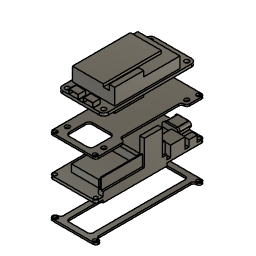
Air_Sensor_Frame (Autodesk Fusion 360 design; units mm, degrees)
Autodesk Fusion 360 part; units mm, degrees
sketch "Sketch1" plane through (0, 0, 0) normal (0, 0, 1) x (1, 0, 0)
  line L0 (-5.5, 4) -> (16.9, 4)
  line L1 (18.4, 2.5) -> (18.4, -54.5)
  line L2 (16.9, -56) -> (-5.5, -56)
  line L3 (-7, -54.5) -> (-7, 2.5)
  line L4 (17.9, 2.5) -> (17.9, 2.5002)
  circle A0 centre (-5.5, 2.5) radius 1
  circle A1 centre (16.9, 2.5) radius 1
  circle A2 centre (16.9, -54.5) radius 1
  circle A3 centre (-5.5, -54.5) radius 1
  line L5 (17.9, 2.5002) -> (17.9, 2.4998)
  arc A4 (-5.5, 4) -> (-7, 2.5) centre (-5.5, 2.5) ccw
  arc A5 (18.4, 2.5) -> (16.9, 4) centre (16.9, 2.5) ccw
  arc A6 (16.9, -56) -> (18.4, -54.5) centre (16.9, -54.5) ccw
  arc A7 (-7, -54.5) -> (-5.5, -56) centre (-5.5, -54.5) ccw
  point P0 (18.4, 4)
  point P1 (-7, -56)
  dimension "d9" = 1.5
  dimension "d10" = 1.5
  dimension "d11" = 1.5
  dimension "d12" = 1.5
  constraint horizontal L0
  constraint vertical L1
  constraint horizontal L2
  constraint vertical L3
  constraint vertical L5
  constraint vertical L4
  constraint coincident A1 L4.end
  constraint coincident A1 L5.end
  constraint tangent L0 A4
  constraint tangent L3 A4
  constraint coincident P0 L0
  constraint coincident P0 L1
  constraint tangent L0 A5
  constraint tangent L1 A5
  constraint tangent L1 A6
  constraint tangent L2 A6
  constraint coincident P1 L3
  constraint coincident P1 L2
  constraint tangent L3 A7
  constraint tangent L2 A7
  measures "d9" radius of A4
  measures "d10" radius of A5
  measures "d11" radius of A6
  measures "d12" radius of A7
extrude "Extrude1" add sketch "Sketch1" along normal blind 1.5 makes body 1
sketch "Sketch2" plane through (0, 0, 1.5) normal (0, 0, 1) x (-1, 0, 0)
  circle A0 centre (5.5, 54.5) radius 1
  circle A1 centre (5.5, -2.5) radius 1
  arc A2 (-17.9, -2.5002) -> (-17.9, -2.4998) centre (-16.9, -2.5) ccw
  line L0 (-17.9, -2.5002) -> (-17.9, -2.4998)
  circle A3 centre (-16.9, 54.5) radius 1
  arc A4 (5.5, -4) -> (7, -2.5) centre (5.5, -2.5) ccw
  line L1 (7, -2.5) -> (7, 54.5)
  arc A5 (7, 54.5) -> (5.5, 56) centre (5.5, 54.5) ccw
  line L2 (5.5, 56) -> (-16.9, 56)
  arc A6 (-16.9, 56) -> (-18.4, 54.5) centre (-16.9, 54.5) ccw
  line L3 (-18.4, 54.5) -> (-18.4, -2.5)
  arc A7 (-18.4, -2.5) -> (-16.9, -4) centre (-16.9, -2.5) ccw
  line L4 (-16.9, -4) -> (5.5, -4)
  line L5 (-1.2, -4) -> (-1.2, -5)
  line L6 (-1.2, -5) -> (-10.2, -5)
  line L7 (-1.2, -4) -> (-1.2, 2.2)
  line L8 (-1.2, 2.2) -> (-10.2, 2.2)
  line L9 (-10.2, 2.2) -> (-10.2, -4)
  line L10 (-10.2, -5) -> (-10.2, -4)
  dimension "d16" = 9
  dimension "d17" = 1
  dimension "d18" = 6.2
  constraint coincident L4 L9.end
  constraint perpendicular L4 L5
  constraint perpendicular L5 L6
  constraint perpendicular L4 L7
  constraint perpendicular L7 L8
  constraint perpendicular L4 L9
  constraint perpendicular L4 L10
  measures "d16" distance of L5.start L9.end
  measures "d17" distance of L5.start L5.end
  measures "d18" distance of L5.start L7.end
extrude "Extrude2" add sketch "Sketch2" along normal blind 3 contours L4 L5 L6 L10 | L4 L7 L8 L9 bodies 1
fillet "Fillet1" radius 1.5 4 edges at (10.2, 1.4, 4.5) (1.2, 1.4, 4.5) (10.2, 4.5, 1.5) (1.2, 4.5, 1.5) on bodies 1
sketch "Sketch3" plane through (0, 5, 0) normal (0, 1, 0) x (-1, 0, 0)
  arc A0 (-2.7, 1.5) -> (-2.7, 4.5) centre (-2.7, 3) ccw
  line L0 (-2.7, 4.5) -> (-8.7, 4.5)
  arc A1 (-8.7, 4.5) -> (-8.7, 1.5) centre (-8.7, 3) ccw
  line L1 (-8.7, 1.5) -> (-2.7, 1.5)
  line L2 (-8.75, 4.4) -> (-2.65, 4.4)
  line L3 (-1.3, 3.05) -> (-1.3, 2.95)
  line L4 (-2.65, 1.6) -> (-8.75, 1.6)
  line L5 (-10.1, 2.95) -> (-10.1, 3.05)
  arc A2 (-8.75, 4.4) -> (-10.1, 3.05) centre (-8.75, 3.05) ccw
  arc A3 (-10.1, 2.95) -> (-8.75, 1.6) centre (-8.75, 2.95) ccw
  arc A4 (-2.65, 1.6) -> (-1.3, 2.95) centre (-2.65, 2.95) ccw
  arc A5 (-1.3, 3.05) -> (-2.65, 4.4) centre (-2.65, 3.05) ccw
  dimension "d23" = 1.35
  constraint horizontal L2
  constraint vertical L3
  constraint horizontal L4
  constraint vertical L5
  constraint tangent L2 A2
  constraint tangent L5 A2
  constraint tangent L4 A3
  constraint tangent L5 A3
  constraint equal A2 A3
  constraint tangent L3 A4
  constraint tangent L4 A4
  constraint equal A2 A4
  constraint tangent L2 A5
  constraint tangent L3 A5
  constraint equal A2 A5
  measures "d23" radius of A2
extrude "Extrude3" cut sketch "Sketch3" against normal blind 6.1 contours L2 L3 L4 L5 A2 A3 A4 A5 bodies 1
sketch "Sketch4" plane through (0, 0, 1.5) normal (0, 0, 1) x (-1, 0, 0)
  line L0 (-1.2, 2.2) -> (-1.2, -4)
  line L1 (-1.2, -4) -> (5.5, -4)
  arc A0 (5.5, -4) -> (7, -2.5) centre (5.5, -2.5) ccw
  line L2 (7, -2.5) -> (7, 54.5)
  arc A1 (7, 54.5) -> (5.5, 56) centre (5.5, 54.5) ccw
  line L3 (5.5, 56) -> (-16.9, 56)
  arc A2 (-16.9, 56) -> (-18.4, 54.5) centre (-16.9, 54.5) ccw
  line L4 (-18.4, 54.5) -> (-18.4, -2.5)
  arc A3 (-18.4, -2.5) -> (-16.9, -4) centre (-16.9, -2.5) ccw
  line L5 (-16.9, -4) -> (-10.2, -4)
  line L6 (-10.2, -4) -> (-10.2, 2.2)
  line L7 (-10.2, 2.2) -> (-1.2, 2.2)
  circle A4 centre (5.5, 54.5) radius 1
  circle A5 centre (5.5, -2.5) radius 1
  arc A6 (-17.9, -2.5002) -> (-17.9, -2.4998) centre (-16.9, -2.5) ccw
  line L8 (-17.9, -2.5002) -> (-17.9, -2.4998)
  circle A7 centre (-16.9, 54.5) radius 1
  line L9 (-18.4, 56) -> (-18.4, 52)
  line L10 (-18.4, 52) -> (-15.9, 52)
  line L11 (-15.9, 52) -> (-15.9, 16.7)
  line L12 (-15.9, 16.7) -> (-18.4, 16.7)
  line L13 (-18.4, 52) -> (-18.4, 16.7)
  dimension "d26" = 4
  dimension "d27" = 2.5
  dimension "d28" = 35.3
  constraint perpendicular L3 L9
  constraint perpendicular L9 L10
  constraint perpendicular L10 L11
  constraint coincident L4 L12.end
  constraint perpendicular L4 L12
  constraint perpendicular L12 L13
  measures "d26" distance of L9.start L9.end
  measures "d27" distance of L9.end L10.end
  measures "d28" distance of L10.end L11.end
extrude "Extrude4" add sketch "Sketch4" along normal blind 2.5 contours L4 L10 L11 L12 L13 bodies 1
sketch "Sketch5" plane through (0, 0, 4) normal (0, 0, 1) x (-1, 0, 0)
  line L0 (-15.9, 52) -> (-18.4, 52)
  line L1 (-18.4, 52) -> (-18.4, 16.7)
  line L2 (-18.4, 16.7) -> (-15.9, 16.7)
  line L3 (-15.9, 16.7) -> (-15.9, 52)
  line L4 (-17.15, 16.7) -> (-16.9, 16.7)
  line L5 (-17.15, 16.7) -> (-17.4, 16.7)
  line L6 (-16.9, 16.7) -> (-17.4, 16.7)
  line L7 (-17.4, 52) -> (-16.9, 52)
  line L8 (-18.4, 16.7) -> (-15.9, 16.7)
  line L9 (-15.9, 16.7) -> (-15.9, 19.2)
  line L10 (-15.9, 19.2) -> (-18.4, 19.2)
  line L11 (-18.4, 19.2) -> (-18.4, 16.7)
  line L12 (-18.4, 19.2) -> (-15.9, 19.2)
  line L13 (-15.9, 19.2) -> (-15.9, 29.2)
  line L14 (-15.9, 29.2) -> (-18.4, 29.2)
  line L15 (-18.4, 29.2) -> (-18.4, 19.2)
  line L16 (-17.4, 16.7) -> (-17.4, 19.2)
  line L17 (-17.4, 29.2) -> (-17.4, 52)
  line L18 (-16.9, 52) -> (-16.9, 29.2)
  line L19 (-16.9, 19.2) -> (-16.9, 16.7)
  dimension "d31" = 0.5
  dimension "d32" = 2.5
  dimension "d33" = 10
  constraint midpoint L2 L4.start
  constraint coincident L2 L4.end
  constraint parallel L2 L4
  constraint coincident L2 L5.end
  constraint parallel L2 L5
  constraint horizontal L6
  constraint vertical L16
  constraint horizontal L7
  constraint vertical L18
  constraint coincident L0 L7.start
  constraint horizontal L8
  constraint vertical L9
  constraint horizontal L10
  constraint vertical L11
  constraint coincident L1.end L2.start
  constraint horizontal L12
  constraint vertical L13
  constraint horizontal L14
  constraint vertical L15
  constraint coincident L10 L16.end
  constraint coincident L14 L17.start
  constraint collinear L16 L17
  constraint coincident L14 L18.end
  constraint coincident L10 L19.start
  constraint collinear L18 L19
  measures "d31" distance of L4.end L5.end
  measures "d32" distance of L1.end L10.end
  measures "d33" distance of L10.end L14.end
extrude "Extrude5" add sketch "Sketch5" along normal blind 6 contours L0 L7 L14 L17 L18 | L2 L4 L5 L6 L8 L10 L12 L16 L19 bodies 1
extrude "Extrude6" add sketch "Sketch5" along normal blind 14 contours L1 L3 L10 L12 L13 L14 L15 bodies 1
sketch "Sketch6" plane through (0, 0, 1.5) normal (0, 0, 1) x (-1, 0, 0)
  line L0 (-15.9, 16.7) -> (-18.4, 16.7)
  line L1 (-18.4, 16.7) -> (-18.4, -2.5)
  arc A0 (-18.4, -2.5) -> (-16.9, -4) centre (-16.9, -2.5) ccw
  line L2 (-16.9, -4) -> (-10.2, -4)
  line L3 (-10.2, -4) -> (-10.2, 2.2)
  line L4 (-10.2, 2.2) -> (-1.2, 2.2)
  line L5 (-1.2, 2.2) -> (-1.2, -4)
  line L6 (-1.2, -4) -> (5.5, -4)
  arc A1 (5.5, -4) -> (7, -2.5) centre (5.5, -2.5) ccw
  line L7 (7, -2.5) -> (7, 54.5)
  arc A2 (7, 54.5) -> (5.5, 56) centre (5.5, 54.5) ccw
  line L8 (5.5, 56) -> (-16.9, 56)
  arc A3 (-16.9, 56) -> (-18.4, 54.5) centre (-16.9, 54.5) ccw
  line L9 (-18.4, 54.5) -> (-18.4, 52)
  line L10 (-18.4, 52) -> (-15.9, 52)
  line L11 (-15.9, 52) -> (-15.9, 16.7)
  circle A4 centre (5.5, 54.5) radius 1
  circle A5 centre (5.5, -2.5) radius 1
  arc A6 (-17.9, -2.5002) -> (-17.9, -2.4998) centre (-16.9, -2.5) ccw
  line L12 (-17.9, -2.5002) -> (-17.9, -2.4998)
  circle A7 centre (-16.9, 54.5) radius 1
  line L13 (-18.4, 16.7) -> (-18.4, 14.7)
  line L14 (-18.4, 14.7) -> (-10.9, 14.7)
  line L15 (-10.9, 14.7) -> (-10.9, 6.7)
  line L16 (-10.9, 6.7) -> (-18.4, 6.7)
  line L17 (-18.4, 6.7) -> (-18.4, 14.7)
  dimension "d38" = 2
  dimension "d39" = 7.5
  dimension "d40" = 8
  constraint coincident L0.end L1.start
  constraint coincident L1 L13.end
  constraint horizontal L14
  constraint vertical L15
  constraint horizontal L16
  constraint vertical L17
  measures "d38" distance of L0.end L13.end
  measures "d39" distance of L13.end L14.end
  measures "d40" distance of L13.end L16.end
extrude "Extrude7" add sketch "Sketch6" along normal blind 6 contours L1 L14 L15 L16 L17 bodies 1
sketch "Sketch7" plane through (0, 0, 1.5) normal (0, 0, 1) x (-1, 0, 0)
  circle A0 centre (-16.9, 54.5) radius 1
  arc A1 (-17.9, -2.5002) -> (-17.9, -2.4998) centre (-16.9, -2.5) ccw
  line L0 (-17.9, -2.5002) -> (-17.9, -2.4998)
  circle A2 centre (5.5, -2.5) radius 1
  circle A3 centre (5.5, 54.5) radius 1
  line L1 (-18.4, 14.7) -> (-10.9, 14.7)
  line L2 (-10.9, 14.7) -> (-10.9, 6.7)
  line L3 (-10.9, 6.7) -> (-18.4, 6.7)
  line L4 (-18.4, 6.7) -> (-18.4, -2.5)
  arc A4 (-18.4, -2.5) -> (-16.9, -4) centre (-16.9, -2.5) ccw
  line L5 (-16.9, -4) -> (-10.2, -4)
  line L6 (-10.2, -4) -> (-10.2, 2.2)
  line L7 (-10.2, 2.2) -> (-1.2, 2.2)
  line L8 (-1.2, 2.2) -> (-1.2, -4)
  line L9 (-1.2, -4) -> (5.5, -4)
  arc A5 (5.5, -4) -> (7, -2.5) centre (5.5, -2.5) ccw
  line L10 (7, -2.5) -> (7, 54.5)
  arc A6 (7, 54.5) -> (5.5, 56) centre (5.5, 54.5) ccw
  line L11 (5.5, 56) -> (-16.9, 56)
  arc A7 (-16.9, 56) -> (-18.4, 54.5) centre (-16.9, 54.5) ccw
  line L12 (-18.4, 54.5) -> (-18.4, 52)
  line L13 (-18.4, 52) -> (-15.9, 52)
  line L14 (-15.9, 52) -> (-15.9, 16.7)
  line L15 (-15.9, 16.7) -> (-18.4, 16.7)
  line L16 (-18.4, 16.7) -> (-18.4, 14.7)
  line L17 (7, 56) -> (2, 56)
  line L18 (2, 56) -> (2, 49)
  line L19 (2, 49) -> (7, 49)
  line L20 (7, 49) -> (7, 56)
  line L21 (2, 49) -> (-13, 49)
  line L22 (-13, 49) -> (-13, 31.5)
  line L23 (-13, 31.5) -> (2, 31.5)
  line L24 (2, 31.5) -> (2, 49)
  line L25 (-5.5, 31.5) -> (-5.5, 28.2)
  line L26 (-5.5, 28.2) -> (2, 28.2)
  line L27 (2, 28.2) -> (2, 26.2)
  line L28 (2, 26.2) -> (-13, 26.2)
  line L29 (-13, 26.2) -> (-13, 28.2)
  line L30 (-13, 28.2) -> (-5.5, 28.2)
  dimension "d43" = 5
  dimension "d44" = 7
  dimension "d45" = 15
  dimension "d46" = 17.5
  dimension "d47" = 3.3
  dimension "d48" = 2
  constraint horizontal L17
  constraint vertical L18
  constraint horizontal L19
  constraint vertical L20
  constraint horizontal L21
  constraint vertical L22
  constraint horizontal L23
  constraint vertical L24
  constraint midpoint L23 L25.start
  constraint perpendicular L23 L25
  constraint perpendicular L25 L26
  constraint perpendicular L26 L27
  constraint perpendicular L25 L28
  constraint perpendicular L26 L29
  constraint perpendicular L25 L30
  measures "d43" distance of L17.start L17.end
  measures "d44" distance of L17.start L19.end
  measures "d45" distance of L18.end L21.end
  measures "d46" distance of L18.end L23.end
  measures "d47" distance of L25.start L25.end
  measures "d48" distance of L26.end L27.end
extrude "Extrude8" add sketch "Sketch7" along normal blind 4 contours L21 L22 L23 L24 bodies 1
extrude "Extrude9" add sketch "Sketch7" along normal blind 5 contours L26 L27 L28 L29 L30 bodies 1
sketch "Sketch8" plane through (0, 0, 1.5) normal (0, 0, 1) x (-1, 0, 0)
  line L0 (-13, 28.2) -> (2, 28.2)
  line L1 (2, 28.2) -> (2, 26.2)
  line L2 (2, 26.2) -> (-13, 26.2)
  line L3 (-13, 26.2) -> (-13, 28.2)
  line L4 (2, 31.5) -> (-13, 31.5)
  line L5 (-13, 31.5) -> (-13, 49)
  line L6 (-13, 49) -> (2, 49)
  line L7 (2, 49) -> (2, 31.5)
  circle A0 centre (-16.9, 54.5) radius 1
  arc A1 (-17.9, -2.5002) -> (-17.9, -2.4998) centre (-16.9, -2.5) ccw
  line L8 (-17.9, -2.5002) -> (-17.9, -2.4998)
  circle A2 centre (5.5, -2.5) radius 1
  circle A3 centre (5.5, 54.5) radius 1
  line L9 (-18.4, 14.7) -> (-10.9, 14.7)
  line L10 (-10.9, 14.7) -> (-10.9, 6.7)
  line L11 (-10.9, 6.7) -> (-18.4, 6.7)
  line L12 (-18.4, 6.7) -> (-18.4, -2.5)
  arc A4 (-18.4, -2.5) -> (-16.9, -4) centre (-16.9, -2.5) ccw
  line L13 (-16.9, -4) -> (-10.2, -4)
  line L14 (-10.2, -4) -> (-10.2, 2.2)
  line L15 (-10.2, 2.2) -> (-1.2, 2.2)
  line L16 (-1.2, 2.2) -> (-1.2, -4)
  line L17 (-1.2, -4) -> (5.5, -4)
  arc A5 (5.5, -4) -> (7, -2.5) centre (5.5, -2.5) ccw
  line L18 (7, -2.5) -> (7, 54.5)
  arc A6 (7, 54.5) -> (5.5, 56) centre (5.5, 54.5) ccw
  line L19 (5.5, 56) -> (-16.9, 56)
  arc A7 (-16.9, 56) -> (-18.4, 54.5) centre (-16.9, 54.5) ccw
  line L20 (-18.4, 54.5) -> (-18.4, 52)
  line L21 (-18.4, 52) -> (-15.9, 52)
  line L22 (-15.9, 52) -> (-15.9, 16.7)
  line L23 (-15.9, 16.7) -> (-18.4, 16.7)
  line L24 (-18.4, 16.7) -> (-18.4, 14.7)
  line L25 (7, -4) -> (4, -4)
  line L26 (4, -4) -> (4, 0)
  line L27 (4, 0) -> (7, 0)
  line L28 (7, 0) -> (7, -4)
  line L29 (-18.4, -4) -> (-15.4, -4)
  line L30 (-15.4, -4) -> (-15.4, 0)
  line L31 (-15.4, 0) -> (-18.4, 0)
  line L32 (-18.4, 0) -> (-18.4, -4)
  line L33 (-15.4, 0) -> (-18.4, 0)
  line L34 (-18.4, 0) -> (-18.4, 4.5)
  line L35 (-18.4, 4.5) -> (-15.4, 4.5)
  line L36 (-15.4, 4.5) -> (-15.4, 0)
  line L37 (4, 0) -> (7, 0)
  line L38 (7, 0) -> (7, 4.5)
  line L39 (7, 4.5) -> (4, 4.5)
  line L40 (4, 4.5) -> (4, 0)
  dimension "d53" = 3
  dimension "d54" = 4
  dimension "d55" = 3
  dimension "d56" = 4
  dimension "d57" = 4.5
  dimension "d58" = 4.5
  constraint horizontal L25
  constraint vertical L26
  constraint horizontal L27
  constraint vertical L28
  constraint horizontal L29
  constraint vertical L30
  constraint horizontal L31
  constraint vertical L32
  constraint horizontal L33
  constraint vertical L34
  constraint horizontal L35
  constraint vertical L36
  constraint horizontal L37
  constraint vertical L38
  constraint horizontal L39
  constraint vertical L40
  measures "d53" distance of L25.start L25.end
  measures "d54" distance of L25.start L27.end
  measures "d55" distance of L29.start L29.end
  measures "d56" distance of L29.start L31.end
  measures "d57" distance of L30.end L35.end
  measures "d58" distance of L26.end L39.end
extrude "Extrude10" add sketch "Sketch8" along normal blind 3.5 contours L12 L31 L33 L34 L35 L36 | L18 L27 L37 L38 L39 L40 bodies 1
sketch "Sketch9" plane through (0, 0, 0) normal (0, 0, 1) x (1, 0, 0)
  line L0 (26, 4) -> (51.3, 4)
  line L1 (51.3, 4) -> (51.3, -47)
  line L2 (51.3, -47) -> (26, -47)
  line L3 (26, -47) -> (26, 4)
  dimension "d61" = 25.3
  dimension "d62" = 51
  constraint horizontal L0
  constraint vertical L1
  constraint horizontal L2
  constraint vertical L3
  measures "d61" distance of L0.start L0.end
  measures "d62" distance of L0.start L2.end
extrude "Extrude11" add sketch "Sketch9" along normal blind 1.5 separate body makes body 2
sketch "Sketch10" plane through (0, 0, 1.5) normal (0, 0, 1) x (-1, 0, 0)
  line L0 (-26, 47) -> (-51.3, 47)
  line L1 (-51.3, 47) -> (-51.3, -4)
  line L2 (-51.3, -4) -> (-26, -4)
  line L3 (-26, -4) -> (-26, 47)
  circle A0 centre (-28.6, -1.4) radius 1.25
  circle A1 centre (-48.7, -1.4) radius 1.25
  circle A2 centre (-28.6, 44.4) radius 1.25
  circle A3 centre (-48.7, 44.4) radius 1.25
  dimension "d69" = 2.5
  dimension "d70" = 2.5
  dimension "d75" = 2.5
  dimension "d76" = 2.5
  measures "d69" diameter of A0
  measures "d70" diameter of A1
  measures "d75" diameter of A2
  measures "d76" diameter of A3
extrude "Extrude12" cut sketch "Sketch10" against normal blind 10 contours A0 | A1 | A2 | A3 bodies 2
fillet "Fillet2" radius 2.5 4 edges at (51.3, -47, 0.75) (26, -47, 0.75) (26, 4, 0.75) (51.3, 4, 0.75) on bodies 2
sketch "Sketch11" plane through (0, 0, 0) normal (0, 0, -1) x (1, 0, 0)
  circle A0 centre (-5.5, 54.5) radius 1
  circle A1 centre (-5.5, -2.5) radius 1
  arc A2 (17.9, -2.4998) -> (17.9, -2.5002) centre (16.9, -2.5) ccw
  line L0 (17.9, -2.4998) -> (17.9, -2.5002)
  circle A3 centre (16.9, 54.5) radius 1
  arc A4 (-7, -2.5) -> (-5.5, -4) centre (-5.5, -2.5) ccw
  line L1 (-5.5, -4) -> (16.9, -4)
  arc A5 (16.9, -4) -> (18.4, -2.5) centre (16.9, -2.5) ccw
  line L2 (18.4, -2.5) -> (18.4, 54.5)
  arc A6 (18.4, 54.5) -> (16.9, 56) centre (16.9, 54.5) ccw
  line L3 (16.9, 56) -> (-5.5, 56)
  arc A7 (-5.5, 56) -> (-7, 54.5) centre (-5.5, 54.5) ccw
  line L4 (-7, 54.5) -> (-7, -2.5)
  line L5 (18.35, 16.7) -> (15.9, 16.7)
  line L6 (15.9, 16.7) -> (15.9, 52)
  line L7 (15.9, 52) -> (18.35, 52)
  line L8 (18.35, 52) -> (18.4, 52)
  line L9 (18.4, 52) -> (18.4, 16.7)
  line L10 (18.35, 16.7) -> (18.4, 16.7)
  constraint horizontal L5
  constraint vertical L6
  constraint horizontal L7
  constraint coincident L2 L8.end
  constraint perpendicular L2 L8
  constraint coincident L2 L9.end
  constraint perpendicular L2 L10
extrude "Extrude13" add sketch "Sketch11" along normal blind 1.5 contours L2 L5 L6 L7 L8 L9 L10 bodies 1
delete_face "DeleteFace1" 1 faces at (18.4, -40.2333, -0.5) on bodies 1
sketch "Sketch12" plane through (0, 0, 1.5) normal (0, 0, 1) x (-1, 0, 0)
  arc A0 (-51.3, -1.5) -> (-48.8, -4) centre (-48.8, -1.5) ccw
  line L0 (-48.8, -4) -> (-28.5, -4)
  arc A1 (-28.5, -4) -> (-26, -1.5) centre (-28.5, -1.5) ccw
  line L1 (-26, -1.5) -> (-26, 44.5)
  arc A2 (-26, 44.5) -> (-28.5, 47) centre (-28.5, 44.5) ccw
  line L2 (-28.5, 47) -> (-48.8, 47)
  arc A3 (-48.8, 47) -> (-51.3, 44.5) centre (-48.8, 44.5) ccw
  line L3 (-51.3, 44.5) -> (-51.3, -1.5)
  circle A4 centre (-48.7, -1.4) radius 1.25
  circle A5 centre (-48.7, 44.4) radius 1.25
  circle A6 centre (-28.6, -1.4) radius 1.25
  circle A7 centre (-28.6, 44.4) radius 1.25
  line L4 (-50.3, 4) -> (-27, 4)
  line L5 (-27, 4) -> (-27, 40)
  line L6 (-27, 40) -> (-50.3, 40)
  line L7 (-50.3, 40) -> (-50.3, 4)
  constraint horizontal L4
  constraint vertical L5
  constraint horizontal L6
  constraint vertical L7
extrude "Extrude14" add sketch "Sketch12" along normal blind 6 contours L4 L5 L6 L7 bodies 2
sketch "Sketch13" plane through (0, 0, 1.5) normal (0, 0, 1) x (-1, 0, 0)
  line L0 (-50.3, 40) -> (-27, 40)
  line L1 (-27, 40) -> (-27, 4)
  line L2 (-27, 4) -> (-50.3, 4)
  line L3 (-50.3, 4) -> (-50.3, 40)
  arc A0 (-51.3, -1.5) -> (-48.8, -4) centre (-48.8, -1.5) ccw
  line L4 (-48.8, -4) -> (-28.5, -4)
  arc A1 (-28.5, -4) -> (-26, -1.5) centre (-28.5, -1.5) ccw
  line L5 (-26, -1.5) -> (-26, 44.5)
  arc A2 (-26, 44.5) -> (-28.5, 47) centre (-28.5, 44.5) ccw
  line L6 (-28.5, 47) -> (-48.8, 47)
  arc A3 (-48.8, 47) -> (-51.3, 44.5) centre (-48.8, 44.5) ccw
  line L7 (-51.3, 44.5) -> (-51.3, -1.5)
  circle A4 centre (-48.7, -1.4) radius 1.25
  circle A5 centre (-48.7, 44.4) radius 1.25
  circle A6 centre (-28.6, -1.4) radius 1.25
  circle A7 centre (-28.6, 44.4) radius 1.25
  line L8 (-51.3, 47) -> (-45.3, 47)
  line L9 (-26, 47) -> (-32, 47)
  line L10 (-45.3, 47) -> (-40.05, 47)
  line L11 (-32, 47) -> (-37.25, 47)
  line L12 (-45.3, 47) -> (-40, 47)
  line L13 (-40, 47) -> (-40, 43)
  line L14 (-40, 43) -> (-45.3, 43)
  line L15 (-45.3, 43) -> (-45.3, 47)
  line L16 (-37.25, 47) -> (-32, 47)
  line L17 (-32, 47) -> (-32, 43)
  line L18 (-32, 43) -> (-37.25, 43)
  line L19 (-37.25, 43) -> (-37.25, 47)
  dimension "d91" = 6
  dimension "d92" = 6
  dimension "d93" = 5.25
  dimension "d94" = 5.25
  dimension "d95" = 4
  dimension "d96" = 5.25
  dimension "d97" = 4
  constraint coincident L6 L8.end
  constraint perpendicular L7 L8
  constraint perpendicular L5 L9
  constraint parallel L6 L10
  constraint parallel L6 L11
  constraint horizontal L12
  constraint vertical L13
  constraint horizontal L14
  constraint vertical L15
  constraint horizontal L16
  constraint vertical L17
  constraint horizontal L18
  constraint vertical L19
  measures "d91" distance of L8.start L8.end
  measures "d92" distance of L9.start L9.end
  measures "d93" distance of L8.end L10.end
  measures "d94" distance of L9.end L11.end
  measures "d95" distance of L8.end L14.end
  measures "d96" distance of L11.end L9.end
  measures "d97" distance of L11.end L18.end
extrude "Extrude15" add sketch "Sketch13" along normal blind 2.6 contours L6 L10 L12 L13 L14 L15 | L6 L11 L16 L17 L18 L19 bodies 2
sketch "Sketch14" plane through (0, -47, 0) normal (0, -1, 0) x (1, 0, 0)
  line L0 (28.5, 1.5) -> (28.5, 0)
  line L1 (28.5, 0) -> (48.8, 0)
  line L2 (48.8, 0) -> (48.8, 1.5)
  line L3 (48.8, 1.5) -> (45.3, 1.5)
  line L4 (45.3, 1.5) -> (45.3, 4.1)
  line L5 (45.3, 4.1) -> (40, 4.1)
  line L6 (40, 4.1) -> (40, 1.5)
  line L7 (40, 1.5) -> (37.25, 1.5)
  line L8 (37.25, 1.5) -> (37.25, 4.1)
  line L9 (37.25, 4.1) -> (32, 4.1)
  line L10 (32, 4.1) -> (32, 1.5)
  line L11 (32, 1.5) -> (28.5, 1.5)
  line L12 (37.1, 3.95) -> (32.15, 3.95)
  line L13 (32.15, 3.95) -> (32.15, 1.65)
  line L14 (32.15, 1.65) -> (37.1, 1.65)
  line L15 (37.1, 1.65) -> (37.1, 3.95)
  line L16 (40.15, 3.95) -> (45.15, 3.95)
  line L17 (45.15, 3.95) -> (45.15, 1.65)
  line L18 (45.15, 1.65) -> (40.15, 1.65)
  line L19 (40.15, 1.65) -> (40.15, 3.95)
  constraint horizontal L12
  constraint vertical L13
  constraint horizontal L14
  constraint vertical L15
  constraint horizontal L16
  constraint vertical L17
  constraint horizontal L18
  constraint vertical L19
extrude "Extrude16" cut sketch "Sketch14" against normal blind 4 contours L12 L13 L14 L15 | L16 L17 L18 L19 bodies 2
sketch "Sketch15" plane through (0, 0, 7.5) normal (0, 0, 1) x (-1, 0, 0)
  line L0 (-50.3, 40) -> (-50.3, 4)
  line L1 (-50.3, 4) -> (-27, 4)
  line L2 (-27, 4) -> (-27, 40)
  line L3 (-27, 40) -> (-50.3, 40)
  line L4 (-50.3, 40) -> (-47.3, 40)
  line L5 (-47.3, 40) -> (-47.3, 24)
  line L6 (-47.3, 24) -> (-50.3, 24)
  line L7 (-50.3, 24) -> (-50.3, 40)
  line L8 (-27, 40) -> (-44, 40)
  line L9 (-44, 40) -> (-44, 8)
  line L10 (-44, 8) -> (-27, 8)
  line L11 (-27, 8) -> (-27, 40)
  dimension "d102" = 3
  dimension "d103" = 16
  dimension "d104" = 17
  dimension "d105" = 32
  constraint horizontal L4
  constraint vertical L5
  constraint horizontal L6
  constraint vertical L7
  constraint coincident L0.start L3.end
  constraint horizontal L8
  constraint vertical L9
  constraint horizontal L10
  constraint vertical L11
  constraint coincident L2.end L3.start
  measures "d102" distance of L0.start L4.end
  measures "d103" distance of L0.start L6.end
  measures "d104" distance of L2.end L8.end
  measures "d105" distance of L2.end L10.end
extrude "Extrude17" add sketch "Sketch15" along normal blind 3 contours L0 L3 L4 L5 L6 L7 bodies 2
extrude "Extrude18" add sketch "Sketch15" along normal blind 1.5 contours L2 L3 L8 L9 L10 L11 bodies 2
sketch "Sketch16" plane through (0, 0, 0) normal (0, 0, -1) x (1, 0, 0)
  circle A0 centre (48.7, -1.4) radius 1.25
  circle A1 centre (48.7, 44.4) radius 1.25
  circle A2 centre (28.6, -1.4) radius 1.25
  circle A3 centre (28.6, 44.4) radius 1.25
  arc A4 (48.8, -4) -> (51.3, -1.5) centre (48.8, -1.5) ccw
  line L0 (51.3, -1.5) -> (51.3, 44.5)
  arc A5 (51.3, 44.5) -> (48.8, 47) centre (48.8, 44.5) ccw
  line L1 (48.8, 47) -> (28.5, 47)
  arc A6 (28.5, 47) -> (26, 44.5) centre (28.5, 44.5) ccw
  line L2 (26, 44.5) -> (26, -1.5)
  arc A7 (26, -1.5) -> (28.5, -4) centre (28.5, -1.5) ccw
  line L3 (28.5, -4) -> (48.8, -4)
  line L4 (47.3, 40) -> (47.3, 35.9)
  line L5 (50.3, 35.9) -> (50.3, 40)
  line L6 (50.3, 40) -> (47.3, 40)
  line L7 (47.3, 35.9) -> (47.3, 24)
  line L8 (47.3, 24) -> (50.3, 24)
  line L9 (50.3, 24) -> (50.3, 35.9)
  constraint vertical L4
  constraint vertical L5
  constraint perpendicular L4 L6
  constraint vertical L7
  constraint horizontal L8
  constraint vertical L9
extrude "Extrude19" add sketch "Sketch16" along normal blind 2 contours L4 L5 L6 L7 L8 L9 bodies 2
move_body "Move1" bodies 1 2 to x (1, 0, 0) y (0, 1, 0) z (0, 0, 1) at (0, 0, 34)
sketch "Sketch17" plane through (0, 0, 0) normal (0, 0, 1) x (1, 0, 0)
extrude "Extrude20" add sketch "Sketch1" along normal blind 1 separate body makes body 3
sketch "Sketch18" plane through (0, 0, 1) normal (0, 0, 1) x (-1, 0, 0)
  circle A0 centre (-16.9, 54.5) radius 1
  circle A1 centre (5.5, 54.5) radius 1
  circle A2 centre (5.5, -2.5) radius 1
  arc A3 (-17.9, -2.5002) -> (-17.9, -2.4998) centre (-16.9, -2.5) ccw
  line L0 (-17.9, -2.5002) -> (-17.9, -2.4998)
  arc A4 (5.5, -4) -> (7, -2.5) centre (5.5, -2.5) ccw
  line L1 (7, -2.5) -> (7, 54.5)
  arc A5 (7, 54.5) -> (5.5, 56) centre (5.5, 54.5) ccw
  line L2 (5.5, 56) -> (-16.9, 56)
  arc A6 (-16.9, 56) -> (-18.4, 54.5) centre (-16.9, 54.5) ccw
  line L3 (-18.4, 54.5) -> (-18.4, -2.5)
  arc A7 (-18.4, -2.5) -> (-16.9, -4) centre (-16.9, -2.5) ccw
  line L4 (-16.9, -4) -> (5.5, -4)
move_body "Move2" bodies 2 1 to x (1, 0, 0) y (0, 1, 0) z (0, 0, 1) at (0, 73, 0)
sketch "Sketch19" plane through (0, 0, 1) normal (0, 0, 1) x (-1, 0, 0)
  line L0 (7, -1) -> (5.5, -1)
  line L1 (4, 0.5) -> (4, 51.5)
  line L2 (5.5, 53) -> (7, 53)
  line L3 (7, 53) -> (7, -1)
  line L4 (-18.4, -1) -> (-16.9, -1)
  line L5 (-15.4, 0.5) -> (-15.4, 51.5)
  line L6 (-16.9, 53) -> (-18.4, 53)
  line L7 (-18.4, 53) -> (-18.4, -1)
  arc A0 (5.5, 53) -> (4, 51.5) centre (5.5, 51.5) ccw
  arc A1 (4, 0.5) -> (5.5, -1) centre (5.5, 0.5) ccw
  arc A2 (-16.9, -1) -> (-15.4, 0.5) centre (-16.9, 0.5) ccw
  arc A3 (-15.4, 51.5) -> (-16.9, 53) centre (-16.9, 51.5) ccw
  point P0 (4, -1)
  point P1 (-15.4, -1)
  dimension "d114" = 3
  dimension "d115" = 54
  dimension "d116" = 3
  dimension "d117" = 54
  dimension "d118" = 1.5
  constraint horizontal L0
  constraint vertical L1
  constraint horizontal L2
  constraint vertical L3
  constraint horizontal L4
  constraint vertical L5
  constraint horizontal L6
  constraint vertical L7
  constraint tangent L1 A0
  constraint tangent L2 A0
  constraint coincident P0 L0
  constraint coincident P0 L1
  constraint tangent L0 A1
  constraint tangent L1 A1
  constraint equal A0 A1
  constraint coincident P1 L4
  constraint coincident P1 L5
  constraint tangent L4 A2
  constraint tangent L5 A2
  constraint equal A0 A2
  constraint tangent L5 A3
  constraint tangent L6 A3
  constraint equal A0 A3
  measures "d114" distance of L0.start P0
  measures "d115" distance of L0.start L2.end
  measures "d116" distance of L4.start P1
  measures "d117" distance of L4.start L6.end
  measures "d118" radius of A0
extrude "Extrude21" cut sketch "Sketch19" against normal blind 3 bodies 3
fillet "Fillet3" radius 1.5 4 edges at (-7, 1, 0.5) (-7, -53, 0.5) (18.4, -53, 0.5) (18.4, 1, 0.5) on bodies 3
sketch "Sketch20" plane through (0, 0, 1) normal (0, 0, 1) x (-1, 0, 0)
  arc A0 (-16.9, -1) -> (-18.4, -2.5) centre (-16.9, -2.5) ccw
  arc A1 (-18.4, -2.5) -> (-16.9, -4) centre (-16.9, -2.5) ccw
  line L0 (-16.9, -4) -> (5.5, -4)
  arc A2 (5.5, -4) -> (7, -2.5) centre (5.5, -2.5) ccw
  arc A3 (7, -2.5) -> (5.5, -1) centre (5.5, -2.5) ccw
  arc A4 (4, 0.5) -> (5.5, -1) centre (5.5, 0.5) ccw
  line L1 (4, 0.5) -> (4, 51.5)
  arc A5 (5.5, 53) -> (4, 51.5) centre (5.5, 51.5) ccw
  arc A6 (5.5, 53) -> (7, 54.5) centre (5.5, 54.5) ccw
  arc A7 (7, 54.5) -> (5.5, 56) centre (5.5, 54.5) ccw
  line L2 (5.5, 56) -> (-16.9, 56)
  arc A8 (-16.9, 56) -> (-18.4, 54.5) centre (-16.9, 54.5) ccw
  arc A9 (-18.4, 54.5) -> (-16.9, 53) centre (-16.9, 54.5) ccw
  arc A10 (-15.4, 51.5) -> (-16.9, 53) centre (-16.9, 51.5) ccw
  line L3 (-15.4, 51.5) -> (-15.4, 0.5)
  arc A11 (-16.9, -1) -> (-15.4, 0.5) centre (-16.9, 0.5) ccw
  circle A12 centre (-16.9, 54.5) radius 1
  circle A13 centre (5.5, 54.5) radius 1
  circle A14 centre (5.5, -2.5) radius 1
  arc A15 (-17.9, -2.5002) -> (-17.9, -2.4998) centre (-16.9, -2.5) ccw
  line L4 (-17.9, -2.5002) -> (-17.9, -2.4998)
  line L5 (-5.7, -4) -> (-5.7, 56)
  line L6 (4, 53) -> (1, 53)
  line L7 (-15.4, -1) -> (-12.4, -1)
  line L8 (-12.4, -1) -> (1, -1)
  line L9 (1, -1) -> (1, 53)
  line L10 (1, 53) -> (-12.4, 53)
  line L11 (-12.4, 53) -> (-12.4, -1)
  dimension "d123" = 3
  constraint midpoint L0 L5.start
  constraint midpoint L2 L5.end
  constraint perpendicular L1 L6
  constraint perpendicular L3 L7
  constraint horizontal L8
  constraint vertical L9
  constraint horizontal L10
  constraint vertical L11
  measures "d123" distance of L7.start L7.end
extrude "Extrude22" cut sketch "Sketch20" against normal blind 8 contours L5 L8 L10 L11 | L5 L8 L9 L10 bodies 3
fillet "Fillet4" radius 1.5 4 edges at (-1, -53, 0.5) (12.4, -53, 0.5) (-1, 1, 0.5) (12.4, 1, 0.5) on bodies 3
sketch "Sketch21" plane through (0, 0, 1) normal (0, 0, 1) x (-1, 0, 0)
  line L0 (-0.5, -1) -> (-10.9, -1)
  arc A0 (-12.4, 0.5) -> (-10.9, -1) centre (-10.9, 0.5) ccw
  line L1 (-12.4, 0.5) -> (-12.4, 51.5)
  arc A1 (-10.9, 53) -> (-12.4, 51.5) centre (-10.9, 51.5) ccw
  line L2 (-10.9, 53) -> (-0.5, 53)
  arc A2 (1, 51.5) -> (-0.5, 53) centre (-0.5, 51.5) ccw
  line L3 (1, 51.5) -> (1, 0.5)
  arc A3 (-0.5, -1) -> (1, 0.5) centre (-0.5, 0.5) ccw
  arc A4 (-16.9, -1) -> (-18.4, -2.5) centre (-16.9, -2.5) ccw
  arc A5 (-18.4, -2.5) -> (-16.9, -4) centre (-16.9, -2.5) ccw
  line L4 (-16.9, -4) -> (5.5, -4)
  arc A6 (5.5, -4) -> (7, -2.5) centre (5.5, -2.5) ccw
  arc A7 (7, -2.5) -> (5.5, -1) centre (5.5, -2.5) ccw
  arc A8 (4, 0.5) -> (5.5, -1) centre (5.5, 0.5) ccw
  line L5 (4, 0.5) -> (4, 51.5)
  arc A9 (5.5, 53) -> (4, 51.5) centre (5.5, 51.5) ccw
  arc A10 (5.5, 53) -> (7, 54.5) centre (5.5, 54.5) ccw
  arc A11 (7, 54.5) -> (5.5, 56) centre (5.5, 54.5) ccw
  line L6 (5.5, 56) -> (-16.9, 56)
  arc A12 (-16.9, 56) -> (-18.4, 54.5) centre (-16.9, 54.5) ccw
  arc A13 (-18.4, 54.5) -> (-16.9, 53) centre (-16.9, 54.5) ccw
  arc A14 (-15.4, 51.5) -> (-16.9, 53) centre (-16.9, 51.5) ccw
  line L7 (-15.4, 51.5) -> (-15.4, 0.5)
  arc A15 (-16.9, -1) -> (-15.4, 0.5) centre (-16.9, 0.5) ccw
  circle A16 centre (-16.9, 54.5) radius 1
  circle A17 centre (5.5, 54.5) radius 1
  circle A18 centre (5.5, -2.5) radius 1
  arc A19 (-17.9, -2.5002) -> (-17.9, -2.4998) centre (-16.9, -2.5) ccw
  line L8 (-17.9, -2.5002) -> (-17.9, -2.4998)
  circle A20 centre (5, -2.5) radius 1
  circle A21 centre (-16.5, -2.5) radius 1
  dimension "d128" = 2
  measures "d128" diameter of A21
extrude "Extrude23" cut sketch "Sketch21" against normal blind 2.5 contours A18 A20 | A19 A21 picked at (4.3378, -2.5729) picked at (-15.6545, -2.3084) bodies 3
fillet "Fillet5" radius 226.05 1 edges at (-5.25, 3.4682, 0.5) on bodies 3
fillet "Fillet6" radius 339 1 edges at (-5.25, 1.5318, 0.5) on bodies 3
fillet "Fillet7" radius 1536 1 edges at (16.7, 1.5202, 0.5) on bodies 3
fillet "Fillet8" radius 610.5 1 edges at (16.7, 3.4798, 0.5) on bodies 3
sketch "Sketch22" plane through (0, 0, 1) normal (0, 0, 1) x (-1, 0, 0)
  arc A0 (-16.5003, -3.5) -> (-16.8997, -3.5) centre (-16.6998, -614) ccw
  arc A1 (-17.9, -2.5002) -> (-16.8997, -3.5) centre (-16.9, -2.5) ccw
  line L0 (-17.9, -2.5002) -> (-17.9, -2.4998)
  arc A2 (-16.8999, -1.5) -> (-17.9, -2.4998) centre (-16.9, -2.5) ccw
  arc A3 (-16.8999, -1.5) -> (-16.5001, -1.5) centre (-16.7003, 1534.5) ccw
  arc A4 (-16.5003, -3.5) -> (-16.5001, -1.5) centre (-16.5, -2.5) ccw
  arc A5 (5.0007, -1.5) -> (5.4993, -1.5) centre (5.25, 337.4999) ccw
  arc A6 (5.4989, -3.5) -> (5.4993, -1.5) centre (5.5, -2.5) ccw
  arc A7 (5.4989, -3.5) -> (5.0011, -3.5) centre (5.2499, -229.5499) ccw
  arc A8 (5.0007, -1.5) -> (5.0011, -3.5) centre (5, -2.5) ccw
  line L1 (-0.5, -1) -> (-10.9, -1)
  arc A9 (-12.4, 0.5) -> (-10.9, -1) centre (-10.9, 0.5) ccw
  line L2 (-12.4, 0.5) -> (-12.4, 51.5)
  arc A10 (-10.9, 53) -> (-12.4, 51.5) centre (-10.9, 51.5) ccw
  line L3 (-10.9, 53) -> (-0.5, 53)
  arc A11 (1, 51.5) -> (-0.5, 53) centre (-0.5, 51.5) ccw
  line L4 (1, 51.5) -> (1, 0.5)
  arc A12 (-0.5, -1) -> (1, 0.5) centre (-0.5, 0.5) ccw
  arc A13 (-16.9, -1) -> (-18.4, -2.5) centre (-16.9, -2.5) ccw
  arc A14 (-18.4, -2.5) -> (-16.9, -4) centre (-16.9, -2.5) ccw
  line L5 (-16.9, -4) -> (5.5, -4)
  arc A15 (5.5, -4) -> (7, -2.5) centre (5.5, -2.5) ccw
  arc A16 (7, -2.5) -> (5.5, -1) centre (5.5, -2.5) ccw
  arc A17 (4, 0.5) -> (5.5, -1) centre (5.5, 0.5) ccw
  line L6 (4, 0.5) -> (4, 51.5)
  arc A18 (5.5, 53) -> (4, 51.5) centre (5.5, 51.5) ccw
  arc A19 (5.5, 53) -> (7, 54.5) centre (5.5, 54.5) ccw
  arc A20 (7, 54.5) -> (5.5, 56) centre (5.5, 54.5) ccw
  line L7 (5.5, 56) -> (-16.9, 56)
  arc A21 (-16.9, 56) -> (-18.4, 54.5) centre (-16.9, 54.5) ccw
  arc A22 (-18.4, 54.5) -> (-16.9, 53) centre (-16.9, 54.5) ccw
  arc A23 (-15.4, 51.5) -> (-16.9, 53) centre (-16.9, 51.5) ccw
  line L8 (-15.4, 51.5) -> (-15.4, 0.5)
  arc A24 (-16.9, -1) -> (-15.4, 0.5) centre (-16.9, 0.5) ccw
  circle A25 centre (-16.9, 54.5) radius 1
  circle A26 centre (5.5, 54.5) radius 1
  line L9 (5, 55) -> (5, 53.9)
  circle A27 centre (5, 54.5) radius 1
  circle A28 centre (-16.5, 54.5) radius 1
  dimension "d139" = 2
  dimension "d140" = 2
  constraint vertical L9
  constraint coincident L9 A27.centre
  measures "d139" diameter of A27
  measures "d140" diameter of A28
extrude "Extrude24" cut sketch "Sketch22" against normal blind 4 contours A25 A28 | A26 A27 picked at (-15.6545, 54.3084) picked at (4.3378, 54.5729) bodies 3
fillet "Fillet9" radius 613 4 edges at (16.7, -53.5202, 0.5) (-5.25, -53.5318, 0.5) (-5.25, -55.4682, 0.5) (16.7, -55.4798, 0.5) on bodies 3
copy_body "CopyPasteBodies1" bodies 3 makes body 4
move_body "Move3" bodies 4 to x (1, 0, 0) y (0, 1, 0) z (0, 0, 1) at (30, 0, 0)
move_body "Move4" bodies 2 to x (1, 0, 0) y (0, 1, 0) z (0, 0, 1) at (-2.95, -77.5, 0)
extrude "Extrude25" add 1 faces at (45.4, -17.5, 0.3333) along direction (1, 0, 0) blind 3 on bodies 4 bodies 4
extrude "Extrude26" cut 1 faces at (46.4, -51.5, 0.6667) along direction (0, -1, 0) blind 1.5 on bodies 4 bodies 4
extrude "Extrude27" add 1 faces at (46.4, -51.5, 0.6667) along direction (0, -1, 0) blind 1.5 on bodies 4 bodies 4
delete_face "DeleteFace2" 2 faces at (47.4577, -53.1074, 0.6667) (48.4, -54.4998, 0.3333) on bodies 4
extrude "Extrude28" cut 1 faces at (47.4002, -53, 0.6667) along direction (0, -1, 0) blind 0.4 on bodies 4 bodies 4
extrude "Extrude29" add 1 faces at (47.4002, -53, 0.6667) along direction (0, -1, 0) blind 0.4 on bodies 4 bodies 4
extrude "Extrude30" cut 1 faces at (48.08, -53.4, 0.6667) along direction (0, -1, 0) blind 1.1 on bodies 4 bodies 4
extrude "Extrude31" add 1 faces at (48.08, -53.4, 0.6667) along direction (0, -1, 0) blind 1.1 on bodies 4 bodies 4
extrude "Extrude32" cut 1 faces at (46.4, -0.5, 0.6667) along direction (0, 1, 0) blind 1.5 on bodies 4 bodies 4
extrude "Extrude33" add 1 faces at (46.4, -0.5, 0.6667) along direction (0, 1, 0) blind 1.5 on bodies 4 bodies 4
extrude "Extrude34" cut 1 faces at (47.4002, 1, 0.6667) along direction (0, 1, 0) blind 0.4 on bodies 4 bodies 4
extrude "Extrude35" add 1 faces at (47.4002, 1, 0.6667) along direction (0, 1, 0) blind 0.4 on bodies 4 bodies 4
extrude "Extrude36" cut 1 faces at (48.08, 1.4, 0.6667) along direction (0, 1, 0) blind 1.1 on bodies 4 bodies 4
extrude "Extrude37" add 1 faces at (48.08, 1.4, 0.6667) along direction (0, 1, 0) blind 1.1 on bodies 4 bodies 4
delete_face "DeleteFace3" 1 faces at (41.9856, 0.5351, 0.6667) on bodies 4
delete_face "DeleteFace4" 1 faces at (41.9856, -52.5351, 0.6667) on bodies 4
extrude "Extrude38" cut 1 faces at (42.4, -35, 0.6667) along direction (-1, 0, 0) blind 19 on bodies 4 bodies 4
extrude "Extrude39" add 1 faces at (42.4, -35, 0.6667) along direction (-1, 0, 0) blind 19.5 on bodies 4 bodies 4
extrude "Extrude40" cut 1 faces at (23.9665, -53, 0.3333) along direction (0, -1, 0) blind 0.4 on bodies 4 bodies 4
extrude "Extrude41" add 1 faces at (23.9665, -53, 0.3333) along direction (0, -1, 0) blind 0.4 on bodies 4 bodies 4
extrude "Extrude42" cut 1 faces at (23.0933, -53.4, 0.3333) along direction (0, -1, 0) blind 1.1 on bodies 4 bodies 4
extrude "Extrude43" add 1 faces at (23.0933, -53.4, 0.3333) along direction (0, -1, 0) blind 1.1 on bodies 4 bodies 4
extrude "Extrude44" cut 1 faces at (22.9, -36, 0.6667) along direction (1, 0, 0) blind 0.1 on bodies 4 bodies 4
extrude "Extrude45" cut 1 faces at (23.9998, 1, 0.6667) along direction (0, 1, 0) blind 0.4 on bodies 4 bodies 4
extrude "Extrude46" add 1 faces at (23.9998, 1, 0.6667) along direction (0, 1, 0) blind 0.4 on bodies 4 bodies 4
extrude "Extrude47" cut 1 faces at (23.32, 1.4, 0.6667) along direction (0, 1, 0) blind 1.1 on bodies 4 bodies 4
extrude "Extrude48" add 1 faces at (23.32, 1.4, 0.6667) along direction (0, 1, 0) blind 1.1 on bodies 4 bodies 4
sketch "Sketch23" plane through (0, 0, 1) normal (0, 0, 1) x (-1, 0, 0)
  line L0 (-23, -2.5) -> (-23, 54.5)
  arc A0 (-23, 54.5) -> (-24.5, 56) centre (-24.5, 54.5) ccw
  line L1 (-24.5, 56) -> (-46.9, 56)
  arc A1 (-46.9, 56) -> (-48.4, 54.5) centre (-46.9, 54.5) ccw
  line L2 (-48.4, 54.5) -> (-48.4, -2.5)
  arc A2 (-48.4, -2.5) -> (-46.9, -4) centre (-46.9, -2.5) ccw
  line L3 (-46.9, -4) -> (-24.5, -4)
  arc A3 (-24.5, -4) -> (-23, -2.5) centre (-24.5, -2.5) ccw
  arc A4 (-24.9993, -1.5) -> (-24.5007, -1.5) centre (-24.75, 337.4999) ccw
  arc A5 (-24.5011, -3.5) -> (-24.5007, -1.5) centre (-24.5, -2.5) ccw
  arc A6 (-24.5011, -3.5) -> (-24.9989, -3.5) centre (-24.7501, -229.5499) ccw
  arc A7 (-24.9993, -1.5) -> (-24.9989, -3.5) centre (-25, -2.5) ccw
  arc A8 (-46.5003, -3.5) -> (-46.8997, -3.5) centre (-46.6998, -614) ccw
  arc A9 (-47.9, -2.5002) -> (-46.8997, -3.5) centre (-46.9, -2.5) ccw
  line L4 (-47.9, -2.5002) -> (-47.9, -2.4998)
  arc A10 (-46.8999, -1.5) -> (-47.9, -2.4998) centre (-46.9, -2.5) ccw
  arc A11 (-46.8999, -1.5) -> (-46.5001, -1.5) centre (-46.7003, 1534.5) ccw
  arc A12 (-46.5003, -3.5) -> (-46.5001, -1.5) centre (-46.5, -2.5) ccw
  arc A13 (-24.9996, 55.5) -> (-24.5004, 55.5) centre (-24.7514, 668.4999) ccw
  arc A14 (-24.5004, 53.5) -> (-24.5004, 55.5) centre (-24.5, 54.5) ccw
  arc A15 (-24.5004, 53.5) -> (-24.9996, 53.5) centre (-24.7464, -559.5) ccw
  arc A16 (-24.9996, 55.5) -> (-24.9996, 53.5) centre (-25, 54.5) ccw
  arc A17 (-46.8997, 55.5) -> (-46.5003, 55.5) centre (-46.6982, 668.5) ccw
  arc A18 (-46.5003, 53.5) -> (-46.5003, 55.5) centre (-46.5, 54.5) ccw
  arc A19 (-46.5003, 53.5) -> (-46.8997, 53.5) centre (-46.7045, -559.5) ccw
  arc A20 (-46.8997, 55.5) -> (-46.8997, 53.5) centre (-46.9, 54.5) ccw
  circle A21 centre (-25.65, 48.9) radius 1.25
  circle A22 centre (-25.65, 3.1) radius 1.25
  circle A23 centre (-45.75, 3.1) radius 1.25
  circle A24 centre (-45.75, 48.9) radius 1.25
extrude "Extrude49" cut sketch "Sketch23" against normal blind 7 contours A21 | A22 | A23 | A24 bodies 4
sketch "Sketch24" plane through (0, 0, 1) normal (0, 0, 1) x (-1, 0, 0)
  circle A0 centre (-45.75, 48.9) radius 1.25
  circle A1 centre (-45.75, 3.1) radius 1.25
  circle A2 centre (-25.65, 48.9) radius 1.25
  circle A3 centre (-25.65, 3.1) radius 1.25
  line L0 (-23, -2.5) -> (-23, 54.5)
  arc A4 (-23, 54.5) -> (-24.5, 56) centre (-24.5, 54.5) ccw
  line L1 (-24.5, 56) -> (-46.9, 56)
  arc A5 (-46.9, 56) -> (-48.4, 54.5) centre (-46.9, 54.5) ccw
  line L2 (-48.4, 54.5) -> (-48.4, -2.5)
  arc A6 (-48.4, -2.5) -> (-46.9, -4) centre (-46.9, -2.5) ccw
  line L3 (-46.9, -4) -> (-24.5, -4)
  arc A7 (-24.5, -4) -> (-23, -2.5) centre (-24.5, -2.5) ccw
  arc A8 (-24.9993, -1.5) -> (-24.5007, -1.5) centre (-24.75, 337.4999) ccw
  arc A9 (-24.5011, -3.5) -> (-24.5007, -1.5) centre (-24.5, -2.5) ccw
  arc A10 (-24.5011, -3.5) -> (-24.9989, -3.5) centre (-24.7501, -229.5499) ccw
  arc A11 (-24.9993, -1.5) -> (-24.9989, -3.5) centre (-25, -2.5) ccw
  arc A12 (-46.5003, -3.5) -> (-46.8997, -3.5) centre (-46.6998, -614) ccw
  arc A13 (-47.9, -2.5002) -> (-46.8997, -3.5) centre (-46.9, -2.5) ccw
  line L4 (-47.9, -2.5002) -> (-47.9, -2.4998)
  arc A14 (-46.8999, -1.5) -> (-47.9, -2.4998) centre (-46.9, -2.5) ccw
  arc A15 (-46.8999, -1.5) -> (-46.5001, -1.5) centre (-46.7003, 1534.5) ccw
  arc A16 (-46.5003, -3.5) -> (-46.5001, -1.5) centre (-46.5, -2.5) ccw
  arc A17 (-24.9996, 55.5) -> (-24.5004, 55.5) centre (-24.7514, 668.4999) ccw
  arc A18 (-24.5004, 53.5) -> (-24.5004, 55.5) centre (-24.5, 54.5) ccw
  arc A19 (-24.5004, 53.5) -> (-24.9996, 53.5) centre (-24.7464, -559.5) ccw
  arc A20 (-24.9996, 55.5) -> (-24.9996, 53.5) centre (-25, 54.5) ccw
  arc A21 (-46.8997, 55.5) -> (-46.5003, 55.5) centre (-46.6982, 668.5) ccw
  arc A22 (-46.5003, 53.5) -> (-46.5003, 55.5) centre (-46.5, 54.5) ccw
  arc A23 (-46.5003, 53.5) -> (-46.8997, 53.5) centre (-46.7045, -559.5) ccw
  arc A24 (-46.8997, 55.5) -> (-46.8997, 53.5) centre (-46.9, 54.5) ccw
move_body "Move5" bodies 2 to x (1, 0, 0) y (0, 1, 0) z (0, 0, 1) at (0, 70, 0)
sketch "Sketch25" plane through (0, 0, 1) normal (0, 0, 1) x (1, 0, 0)
  line L0 (25.65, -47.65) -> (25.65, -50.15)
  line L1 (45.75, -1.85) -> (45.75, -4.35)
  line L2 (45.75, -3.1) -> (25.65, -3.1)
  line L3 (25.65, -3.1) -> (25.65, -48.9)
  line L4 (45.75, -48.9) -> (45.75, -3.1)
  line L5 (35.7, -53) -> (30.7, -53)
  line L6 (30.7, -53) -> (40.7, -53)
  line L7 (42.7, -51) -> (42.7, -42)
  line L8 (28.7, -42) -> (28.7, -51)
  line L9 (30.7, -40) -> (40.7, -40)
  line L10 (25.65, -48.9) -> (28.7, -48.9)
  arc A0 (30.7, -40) -> (28.7, -42) centre (30.7, -42) ccw
  arc A1 (42.7, -42) -> (40.7, -40) centre (40.7, -42) ccw
  arc A2 (40.7, -53) -> (42.7, -51) centre (40.7, -51) ccw
  arc A3 (28.7, -51) -> (30.7, -53) centre (30.7, -51) ccw
  point P0 (42.7, -53)
  dimension "d199" = 2
  dimension "d200" = 2
  constraint vertical L0
  constraint vertical L1
  constraint horizontal L2
  constraint vertical L3
  constraint horizontal L10
  constraint vertical L4
  constraint midpoint L0 L3.end
  constraint midpoint L1 L2.start
  constraint horizontal L6
  constraint vertical L7
  constraint vertical L8
  constraint perpendicular L7 L9
  constraint coincident L8 L10.end
  constraint tangent L9 A0
  constraint tangent L8 A0
  constraint tangent L9 A1
  constraint tangent L7 A1
  constraint equal A0 A1
  constraint coincident P0 L6
  constraint coincident P0 L7
  constraint tangent L6 A2
  constraint tangent L7 A2
  constraint equal A0 A2
  constraint tangent L6 A3
  constraint tangent L8 A3
  measures "d199" radius of A0
  measures "d200" radius of A3
extrude "Extrude50" cut sketch "Sketch25" against normal blind 5 bodies 4
sketch "Sketch26" plane through (0, 0, 1) normal (0, 0, 1) x (-1, 0, 0)
  line L0 (-25.65, 4.35) -> (-25.65, 5.75)
  line L1 (-25.65, 5.75) -> (-23, 5.75)
  line L2 (-23, 5.75) -> (-26, 5.75)
  line L3 (-26, 5.75) -> (-26, 40)
  line L4 (-26, 40) -> (-23, 40)
  line L5 (-23, 5.75) -> (-23, 40)
  dimension "d203" = 1.4
  constraint vertical L0
  constraint perpendicular L0 L1
  constraint perpendicular L0 L2
  constraint perpendicular L2 L3
  constraint perpendicular L3 L4
  constraint perpendicular L1 L5
  measures "d203" distance of L0.start L0.end
extrude "Extrude51" cut sketch "Sketch26" against normal blind 4 bodies 4
fillet "Fillet10" radius 1.5 2 edges at (26, -5.75, 0.5) (26, -40, 0.5) on bodies 4
fillet "Fillet11" radius 1.5 2 edges at (23, -5.75, 0.5) (23, -40, 0.5) on bodies 4
sketch "Sketch27" plane through (0, 0, 0) normal (0, 0, 1) x (1, 0, 0)
  line L0 (-95, -61) -> (-31, -61)
  line L1 (-31, -61) -> (-31, -76)
  line L2 (-31, -76) -> (-95, -76)
  line L3 (-95, -76) -> (-95, -61)
  constraint horizontal L0
  constraint vertical L1
  constraint horizontal L2
  constraint vertical L3
move_body "Move9" bodies 1 to x (1, 0, 0) y (0, 1, 0) z (0, 0, 1) at (0, -73, -14)
move_body "Move10" bodies 4 to x (-1, 0, 0) y (0, 1, 0) z (0, 0, -1) at (41.4, 0, 42)
move_body "Move11" bodies 2 to x (1, 0, 0) y (0, 1, 0) z (0, 0, 1) at (-30, -70, 25)
